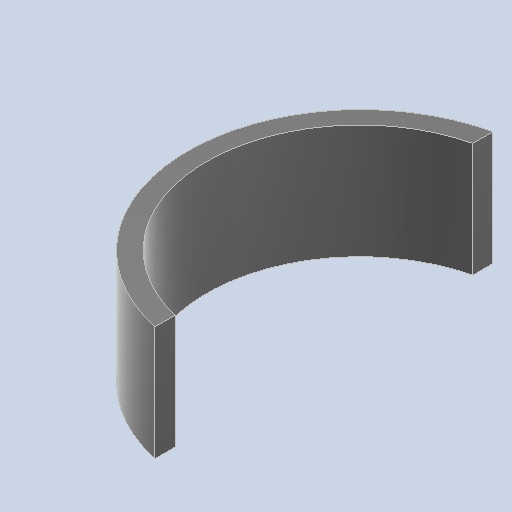
# Autodesk Inventor part: Slicer Strap
Saved by Autodesk Inventor 2022 (Build 260153000, 153)
## iProperties
Created: 2022-03-24
Part Number: Slicer Strap
Material: Thermoplastic Resin
Document SubType Name: Modeling
Designer: mpate
Density: 1.28 g/cm^3
Appearance: Smooth - Black
Author: mpate
Autodesk Inventor part; units mm, degrees
ref_plane "YZ Plane" through (0, 0, 0) normal (1, 0, 0) x (0, 1, 0)
ref_plane "XZ Plane" through (0, 0, 0) normal (0, 1, 0) x (-1, 0, 0)
ref_plane "XY Plane" through (0, 0, 0) normal (0, 0, 1) x (1, 0, 0)
sketch "Sketch1" plane through (0, 0, 0) normal (0, 1, 0) x (-1, 0, 0)
  line L0 (0, 0) -> (0, -151)
  arc A0 (0, -151) -> (0, 0) centre (-16.5983, -75.5) ccw
  arc A1 (0, -142) -> (0, -9) centre (-15.9369, -75.5) ccw
  dimension "d0" = 151
  dimension "d2" = 9
  dimension "d3" = 9
  dimension "d13" = 77.303
  dimension "d14" = 68.383
  constraints: 4 point on circle, 2 centre point, 2 end point, 2 point on line, 1 vertical
  measures "d0" distance of L0.start L0.end
  measures "d2" distance of L0.start A1.end
  measures "d3" distance of L0.end A1.start
  measures "d13" radius of A0
  measures "d14" radius of A1
extrude "Extrusion1" add sketch "Sketch1" along normal blind 51 contours A0 L0 A1
body "Solid1"
